Autodesk Fusion 360 part; units mm, degrees
note: some values were not read from the file. Chosen so that the rebuilt part matches the saved one: which face or edge a step refers to. Set by a fixed rule: which sketch regions a step uses.
(part 7 of 7)
  spline S202 degree 3 poles (37.6254, -69.5482) (37.6638, -69.7473) (37.7012, -69.9549) (37.7371, -70.1712) knots 0 0 0 0 1 1 1 1
  spline S203 degree 3 poles (37.7371, -70.1712) (37.8704, -70.972) (37.9841, -71.8901) (38.0568, -72.9254) knots 0 0 0 0 1 1 1 1
  arc A203 (36.6287, -73.6531) -> (38.0568, -72.9254) centre (0, 0) ccw
  spline S204 degree 3 poles (36.6287, -73.6531) (35.8338, -72.9858) (35.1579, -72.3541) (34.5883, -71.7756) knots 0 0 0 0 1 1 1 1
  spline S205 degree 3 poles (34.5883, -71.7756) (34.4345, -71.6193) (34.2885, -71.4671) (34.15, -71.319) knots 0 0 0 0 1 1 1 1
  arc A204 (34.15, -71.319) -> (33.6869, -71.2307) centre (33.8579, -71.5923) ccw
  arc A205 (32.2864, -71.8764) -> (33.6869, -71.2307) centre (0, 0) ccw
  arc A206 (32.2864, -71.8764) -> (32.0528, -72.2858) centre (32.4503, -72.2413) ccw
  spline S206 degree 3 poles (32.0528, -72.2858) (32.0754, -72.4873) (32.0964, -72.6972) (32.1152, -72.9157) knots 0 0 0 0 1 1 1 1
  spline S207 degree 3 poles (32.1152, -72.9157) (32.1852, -73.7245) (32.2266, -74.6487) (32.2178, -75.6865) knots 0 0 0 0 1 1 1 1
  arc A207 (30.737, -76.2999) -> (32.2178, -75.6865) centre (0, 0) ccw
  spline S208 degree 3 poles (30.737, -76.2999) (29.997, -75.5723) (29.3727, -74.8895) (28.8503, -74.2681) knots 0 0 0 0 1 1 1 1
  spline S209 degree 3 poles (28.8503, -74.2681) (28.7092, -74.1003) (28.5755, -73.937) (28.4491, -73.7785) knots 0 0 0 0 1 1 1 1
  arc A208 (28.4491, -73.7785) -> (27.9944, -73.6542) centre (28.1365, -74.0281) ccw
  arc A209 (26.5475, -74.188) -> (27.9944, -73.6542) centre (0, 0) ccw
  arc A210 (26.5475, -74.188) -> (26.2825, -74.5778) centre (26.6822, -74.5646) ccw
  spline S210 degree 3 poles (26.2825, -74.5778) (26.2892, -74.7805) (26.2937, -74.9914) (26.2953, -75.2107) knots 0 0 0 0 1 1 1 1
  spline S211 degree 3 poles (26.2953, -75.2107) (26.3016, -76.0225) (26.2704, -76.9471) (26.1802, -77.981) knots 0 0 0 0 1 1 1 1
  arc A211 (24.6558, -78.4763) -> (26.1802, -77.981) centre (0, 0) ccw
  spline S212 degree 3 poles (24.6558, -78.4763) (23.9752, -77.6928) (23.4064, -76.9632) (22.9343, -76.3027) knots 0 0 0 0 1 1 1 1
  spline S213 degree 3 poles (22.9343, -76.3027) (22.8068, -76.1243) (22.6864, -75.9511) (22.5728, -75.7832) knots 0 0 0 0 1 1 1 1
  arc A212 (22.5728, -75.7832) -> (22.1292, -75.6235) centre (22.2416, -76.0074) ccw
  arc A213 (20.6449, -76.0422) -> (22.1292, -75.6235) centre (0, 0) ccw
  arc A214 (20.6449, -76.0422) -> (20.3501, -76.41) centre (20.7497, -76.4282) ccw
  spline S214 degree 3 poles (20.3501, -76.41) (20.341, -76.6126) (20.3288, -76.8232) (20.3133, -77.0419) knots 0 0 0 0 1 1 1 1
  spline S215 degree 3 poles (20.3133, -77.0419) (20.2559, -77.8517) (20.1522, -78.771) (19.9812, -79.7947) knots 0 0 0 0 1 1 1 1
  arc A215 (18.4227, -80.1689) -> (19.9812, -79.7947) centre (0, 0) ccw
  spline S216 degree 3 poles (18.4227, -80.1689) (17.8055, -79.3344) (17.2958, -78.5624) (16.877, -77.8669) knots 0 0 0 0 1 1 1 1
  spline S217 degree 3 poles (16.877, -77.8669) (16.7639, -77.6791) (16.6574, -77.4969) (16.5573, -77.3206) knots 0 0 0 0 1 1 1 1
  arc A216 (16.5573, -77.3206) -> (16.1277, -77.1267) centre (16.2095, -77.5182) ccw
  arc A217 (14.6151, -77.4275) -> (16.1277, -77.1267) centre (0, 0) ccw
  arc A218 (14.6151, -77.4275) -> (14.2923, -77.7712) centre (14.6893, -77.8206) ccw
  spline S218 degree 3 poles (14.2923, -77.7712) (14.2673, -77.9723) (14.2387, -78.1814) (14.2061, -78.3982) knots 0 0 0 0 1 1 1 1
  spline S219 degree 3 poles (14.2061, -78.3982) (14.0853, -79.201) (13.9098, -80.1093) (13.659, -81.1164) knots 0 0 0 0 1 1 1 1
  arc A219 (12.0759, -81.3672) -> (13.659, -81.1164) centre (0, 0) ccw
  spline S220 degree 3 poles (12.0759, -81.3672) (11.5261, -80.4868) (11.0785, -79.6772) (10.7156, -78.951) knots 0 0 0 0 1 1 1 1
  spline S221 degree 3 poles (10.7156, -78.951) (10.6176, -78.7549) (10.5258, -78.5649) (10.4398, -78.3813) knots 0 0 0 0 1 1 1 1
  arc A220 (10.4398, -78.3813) -> (10.0267, -78.1543) centre (10.0776, -78.551) ccw
  arc A221 (8.4951, -78.3355) -> (10.0267, -78.1543) centre (0, 0) ccw
  arc A222 (8.4951, -78.3355) -> (8.1464, -78.6528) centre (8.5383, -78.7332) ccw
  spline S222 degree 3 poles (8.1464, -78.6528) (8.1057, -78.8514) (8.0608, -79.0575) (8.0112, -79.2711) knots 0 0 0 0 1 1 1 1
  spline S223 degree 3 poles (8.0112, -79.2711) (7.8278, -80.0619) (7.5816, -80.9537) (7.2526, -81.938) knots 0 0 0 0 1 1 1 1
  arc A223 (5.6547, -82.0638) -> (7.2526, -81.938) centre (0, 0) ccw
  spline S224 degree 3 poles (5.6547, -82.0638) (5.1757, -81.1431) (4.793, -80.3008) (4.4881, -79.5484) knots 0 0 0 0 1 1 1 1
  spline S225 degree 3 poles (4.4881, -79.5484) (4.4058, -79.3452) (4.3292, -79.1486) (4.2579, -78.9588) knots 0 0 0 0 1 1 1 1
  arc A224 (4.2579, -78.9588) -> (3.8638, -78.7) centre (3.8835, -79.0995) ccw
  arc A225 (2.3228, -78.7606) -> (3.8638, -78.7) centre (0, 0) ccw
  arc A226 (2.3228, -78.7606) -> (1.9503, -79.0495) centre (2.3346, -79.1604) ccw
  spline S226 degree 3 poles (1.9503, -79.0495) (1.8941, -79.2443) (1.8331, -79.4462) (1.767, -79.6553) knots 0 0 0 0 1 1 1 1
  spline S227 degree 3 poles (1.767, -79.6553) (1.5221, -80.4293) (1.2067, -81.299) (0.8014, -82.2545) knots 0 0 0 0 1 1 1 1
  arc A227 (-0.8014, -82.2545) -> (0.8014, -82.2545) centre (0, 0) ccw
  spline S228 degree 3 poles (-0.8014, -82.2545) (-1.2067, -81.299) (-1.5221, -80.4293) (-1.767, -79.6553) knots 0 0 0 0 1 1 1 1
  spline S229 degree 3 poles (-1.767, -79.6553) (-1.8331, -79.4462) (-1.8941, -79.2443) (-1.9503, -79.0495) knots 0 0 0 0 1 1 1 1
  arc A228 (-1.9503, -79.0495) -> (-2.3228, -78.7606) centre (-2.3346, -79.1604) ccw
  arc A229 (-3.8638, -78.7) -> (-2.3228, -78.7606) centre (0, 0) ccw
  arc A230 (-3.8638, -78.7) -> (-4.2579, -78.9588) centre (-3.8835, -79.0995) ccw
  spline S230 degree 3 poles (-4.2579, -78.9588) (-4.3292, -79.1486) (-4.4058, -79.3452) (-4.4881, -79.5484) knots 0 0 0 0 1 1 1 1
  spline S231 degree 3 poles (-4.4881, -79.5484) (-4.793, -80.3008) (-5.1757, -81.1431) (-5.6547, -82.0638) knots 0 0 0 0 1 1 1 1
  arc A231 (-7.2526, -81.938) -> (-5.6547, -82.0638) centre (0, 0) ccw
  spline S232 degree 3 poles (-7.2526, -81.938) (-7.5816, -80.9537) (-7.8278, -80.0619) (-8.0112, -79.2711) knots 0 0 0 0 1 1 1 1
  spline S233 degree 3 poles (-8.0112, -79.2711) (-8.0608, -79.0575) (-8.1057, -78.8514) (-8.1464, -78.6528) knots 0 0 0 0 1 1 1 1
  arc A232 (-8.1464, -78.6528) -> (-8.4951, -78.3355) centre (-8.5383, -78.7332) ccw
  arc A233 (-10.0267, -78.1543) -> (-8.4951, -78.3355) centre (0, 0) ccw
  arc A234 (-10.0267, -78.1543) -> (-10.4398, -78.3813) centre (-10.0776, -78.551) ccw
  spline S234 degree 3 poles (-10.4398, -78.3813) (-10.5258, -78.5649) (-10.6176, -78.7549) (-10.7156, -78.951) knots 0 0 0 0 1 1 1 1
  spline S235 degree 3 poles (-10.7156, -78.951) (-11.0785, -79.6772) (-11.5261, -80.4868) (-12.0759, -81.3672) knots 0 0 0 0 1 1 1 1
  arc A235 (-13.659, -81.1164) -> (-12.0759, -81.3672) centre (0, 0) ccw
  spline S236 degree 3 poles (-13.659, -81.1164) (-13.9098, -80.1093) (-14.0853, -79.201) (-14.2061, -78.3982) knots 0 0 0 0 1 1 1 1
  spline S237 degree 3 poles (-14.2061, -78.3982) (-14.2387, -78.1814) (-14.2673, -77.9723) (-14.2923, -77.7712) knots 0 0 0 0 1 1 1 1
  arc A236 (-14.2923, -77.7712) -> (-14.6151, -77.4275) centre (-14.6893, -77.8206) ccw
  arc A237 (-16.1277, -77.1267) -> (-14.6151, -77.4275) centre (0, 0) ccw
  arc A238 (-16.1277, -77.1267) -> (-16.5573, -77.3206) centre (-16.2095, -77.5182) ccw
  spline S238 degree 3 poles (-16.5573, -77.3206) (-16.6574, -77.4969) (-16.7639, -77.6791) (-16.877, -77.8669) knots 0 0 0 0 1 1 1 1
  spline S239 degree 3 poles (-16.877, -77.8669) (-17.2958, -78.5624) (-17.8055, -79.3344) (-18.4227, -80.1689) knots 0 0 0 0 1 1 1 1
  arc A239 (-19.9812, -79.7947) -> (-18.4227, -80.1689) centre (0, 0) ccw
  spline S240 degree 3 poles (-19.9812, -79.7947) (-20.1522, -78.771) (-20.2559, -77.8517) (-20.3133, -77.0419) knots 0 0 0 0 1 1 1 1
  spline S241 degree 3 poles (-20.3133, -77.0419) (-20.3288, -76.8232) (-20.341, -76.6126) (-20.3501, -76.41) knots 0 0 0 0 1 1 1 1
  arc A240 (-20.3501, -76.41) -> (-20.6449, -76.0422) centre (-20.7497, -76.4282) ccw
  arc A241 (-22.1292, -75.6235) -> (-20.6449, -76.0422) centre (0, 0) ccw
  arc A242 (-22.1292, -75.6235) -> (-22.5728, -75.7832) centre (-22.2416, -76.0074) ccw
  spline S242 degree 3 poles (-22.5728, -75.7832) (-22.6864, -75.9511) (-22.8068, -76.1243) (-22.9343, -76.3027) knots 0 0 0 0 1 1 1 1
  spline S243 degree 3 poles (-22.9343, -76.3027) (-23.4064, -76.9632) (-23.9752, -77.6928) (-24.6558, -78.4763) knots 0 0 0 0 1 1 1 1
  arc A243 (-26.1802, -77.981) -> (-24.6558, -78.4763) centre (0, 0) ccw
  spline S244 degree 3 poles (-26.1802, -77.981) (-26.2704, -76.9471) (-26.3016, -76.0225) (-26.2953, -75.2107) knots 0 0 0 0 1 1 1 1
  spline S245 degree 3 poles (-26.2953, -75.2107) (-26.2937, -74.9914) (-26.2892, -74.7805) (-26.2825, -74.5778) knots 0 0 0 0 1 1 1 1
  arc A244 (-26.2825, -74.5778) -> (-26.5475, -74.188) centre (-26.6822, -74.5646) ccw
  arc A245 (-27.9944, -73.6542) -> (-26.5475, -74.188) centre (0, 0) ccw
  arc A246 (-27.9944, -73.6542) -> (-28.4491, -73.7785) centre (-28.1365, -74.0281) ccw
  spline S246 degree 3 poles (-28.4491, -73.7785) (-28.5755, -73.937) (-28.7092, -74.1003) (-28.8503, -74.2681) knots 0 0 0 0 1 1 1 1
  spline S247 degree 3 poles (-28.8503, -74.2681) (-29.3727, -74.8895) (-29.997, -75.5723) (-30.737, -76.2999) knots 0 0 0 0 1 1 1 1
  arc A247 (-32.2178, -75.6865) -> (-30.737, -76.2999) centre (0, 0) ccw
  spline S248 degree 3 poles (-32.2178, -75.6865) (-32.2266, -74.6487) (-32.1852, -73.7245) (-32.1152, -72.9157) knots 0 0 0 0 1 1 1 1
  spline S249 degree 3 poles (-32.1152, -72.9157) (-32.0964, -72.6972) (-32.0754, -72.4873) (-32.0528, -72.2858) knots 0 0 0 0 1 1 1 1
  arc A248 (-32.0528, -72.2858) -> (-32.2864, -71.8764) centre (-32.4503, -72.2413) ccw
  arc A249 (-33.6869, -71.2307) -> (-32.2864, -71.8764) centre (0, 0) ccw
  arc A250 (-33.6869, -71.2307) -> (-34.15, -71.319) centre (-33.8579, -71.5923) ccw
  spline S250 degree 3 poles (-34.15, -71.319) (-34.2885, -71.4671) (-34.4345, -71.6193) (-34.5883, -71.7756) knots 0 0 0 0 1 1 1 1
  spline S251 degree 3 poles (-34.5883, -71.7756) (-35.1579, -72.3541) (-35.8338, -72.9858) (-36.6287, -73.6531) knots 0 0 0 0 1 1 1 1
  arc A251 (-38.0568, -72.9254) -> (-36.6287, -73.6531) centre (0, 0) ccw
  spline S252 degree 3 poles (-38.0568, -72.9254) (-37.9841, -71.8901) (-37.8704, -70.972) (-37.7371, -70.1712) knots 0 0 0 0 1 1 1 1
  spline S253 degree 3 poles (-37.7371, -70.1712) (-37.7012, -69.9549) (-37.6638, -69.7473) (-37.6254, -69.5482) knots 0 0 0 0 1 1 1 1
  arc A252 (-37.6254, -69.5482) -> (-37.8262, -69.1217) centre (-38.0182, -69.4726) ccw
  arc A253 (-39.1718, -68.3681) -> (-37.8262, -69.1217) centre (0, 0) ccw
  arc A254 (-39.1718, -68.3681) -> (-39.6403, -68.4198) centre (-39.3706, -68.7152) ccw
  spline S254 degree 3 poles (-39.6403, -68.4198) (-39.79, -68.5565) (-39.9475, -68.6969) (-40.1132, -68.8406) knots 0 0 0 0 1 1 1 1
  spline S255 degree 3 poles (-40.1132, -68.8406) (-40.7264, -69.3726) (-41.4498, -69.9493) (-42.2945, -70.5522) knots 0 0 0 0 1 1 1 1
  arc A255 (-43.6612, -69.7147) -> (-42.2945, -70.5522) centre (0, 0) ccw
  spline S256 degree 3 poles (-43.6612, -69.7147) (-43.5075, -68.6883) (-43.322, -67.7819) (-43.1264, -66.9941) knots 0 0 0 0 1 1 1 1
  spline S257 degree 3 poles (-43.1264, -66.9941) (-43.0736, -66.7812) (-43.02, -66.5772) (-42.9661, -66.3817) knots 0 0 0 0 1 1 1 1
  arc A256 (-42.9661, -66.3817) -> (-43.1328, -65.9408) centre (-43.3518, -66.2755) ccw
  arc A257 (-44.4151, -65.084) -> (-43.1328, -65.9408) centre (0, 0) ccw
  arc A258 (-44.4151, -65.084) -> (-44.8863, -65.0987) centre (-44.6406, -65.4144) ccw
  spline S258 degree 3 poles (-44.8863, -65.0987) (-45.0463, -65.2233) (-45.2143, -65.3508) (-45.3907, -65.4811) knots 0 0 0 0 1 1 1 1
  spline S259 degree 3 poles (-45.3907, -65.4811) (-46.0437, -65.9633) (-46.8101, -66.4815) (-47.6996, -67.0163) knots 0 0 0 0 1 1 1 1
  arc A259 (-48.9963, -66.0742) -> (-47.6996, -67.0163) centre (0, 0) ccw
  spline S260 degree 3 poles (-48.9963, -66.0742) (-48.7626, -65.063) (-48.5066, -64.174) (-48.2497, -63.4039) knots 0 0 0 0 1 1 1 1
  spline S261 degree 3 poles (-48.2497, -63.4039) (-48.1804, -63.1959) (-48.111, -62.9966) (-48.0419, -62.806) knots 0 0 0 0 1 1 1 1
  arc A260 (-48.0419, -62.806) -> (-48.1735, -62.3533) centre (-48.418, -62.6699) ccw
  arc A261 (-49.3846, -61.3986) -> (-48.1735, -62.3533) centre (0, 0) ccw
  arc A262 (-49.3846, -61.3986) -> (-49.8555, -61.3763) centre (-49.6353, -61.7102) ccw
  spline S262 degree 3 poles (-49.8555, -61.3763) (-50.0247, -61.4879) (-50.2023, -61.6019) (-50.3883, -61.7179) knots 0 0 0 0 1 1 1 1
  spline S263 degree 3 poles (-50.3883, -61.7179) (-51.0772, -62.1475) (-51.8819, -62.6039) (-52.8106, -63.0673) knots 0 0 0 0 1 1 1 1
  arc A263 (-54.0294, -62.0263) -> (-52.8106, -63.0673) centre (0, 0) ccw
  spline S264 degree 3 poles (-54.0294, -62.0263) (-53.717, -61.0366) (-53.3921, -60.1704) (-53.0756, -59.4228) knots 0 0 0 0 1 1 1 1
  spline S265 degree 3 poles (-53.0756, -59.4228) (-52.9901, -59.2209) (-52.9053, -59.0277) (-52.8215, -58.8431) knots 0 0 0 0 1 1 1 1
  arc A264 (-52.8215, -58.8431) -> (-52.9172, -58.3815) centre (-53.1858, -58.6778) ccw
  arc A265 (-54.0497, -57.3346) -> (-52.9172, -58.3815) centre (0, 0) ccw
  arc A266 (-54.0497, -57.3346) -> (-54.5174, -57.2755) centre (-54.324, -57.6257) ccw
  spline S266 degree 3 poles (-54.5174, -57.2755) (-54.6948, -57.3735) (-54.8807, -57.4732) (-55.0753, -57.5742) knots 0 0 0 0 1 1 1 1
  spline S267 degree 3 poles (-55.0753, -57.5742) (-55.7958, -57.9484) (-56.6338, -58.3403) (-57.596, -58.7294) knots 0 0 0 0 1 1 1 1
  arc A267 (-58.7294, -57.596) -> (-57.596, -58.7294) centre (0, 0) ccw
  spline S268 degree 3 poles (-58.7294, -57.596) (-58.3403, -56.6338) (-57.9484, -55.7958) (-57.5742, -55.0753) knots 0 0 0 0 1 1 1 1
  spline S269 degree 3 poles (-57.5742, -55.0753) (-57.4732, -54.8807) (-57.3735, -54.6948) (-57.2755, -54.5174) knots 0 0 0 0 1 1 1 1
  arc A268 (-57.2755, -54.5174) -> (-57.3346, -54.0497) centre (-57.6257, -54.324) ccw
  arc A269 (-58.3815, -52.9172) -> (-57.3346, -54.0497) centre (0, 0) ccw
  arc A270 (-58.3815, -52.9172) -> (-58.8431, -52.8215) centre (-58.6778, -53.1858) ccw
  spline S270 degree 3 poles (-58.8431, -52.8215) (-59.0277, -52.9053) (-59.2209, -52.9901) (-59.4228, -53.0756) knots 0 0 0 0 1 1 1 1
  spline S271 degree 3 poles (-59.4228, -53.0756) (-60.1704, -53.3921) (-61.0366, -53.717) (-62.0263, -54.0294) knots 0 0 0 0 1 1 1 1
  arc A271 (-63.0673, -52.8106) -> (-62.0263, -54.0294) centre (0, 0) ccw
  spline S272 degree 3 poles (-63.0673, -52.8106) (-62.6039, -51.8819) (-62.1475, -51.0772) (-61.7179, -50.3883) knots 0 0 0 0 1 1 1 1
  spline S273 degree 3 poles (-61.7179, -50.3883) (-61.6019, -50.2023) (-61.4879, -50.0247) (-61.3763, -49.8555) knots 0 0 0 0 1 1 1 1
  arc A272 (-61.3763, -49.8555) -> (-61.3986, -49.3846) centre (-61.7102, -49.6353) ccw
  arc A273 (-62.3533, -48.1735) -> (-61.3986, -49.3846) centre (0, 0) ccw
  arc A274 (-62.3533, -48.1735) -> (-62.806, -48.0419) centre (-62.6699, -48.418) ccw
  spline S274 degree 3 poles (-62.806, -48.0419) (-62.9966, -48.111) (-63.1959, -48.1804) (-63.4039, -48.2497) knots 0 0 0 0 1 1 1 1
  spline S275 degree 3 poles (-63.4039, -48.2497) (-64.174, -48.5066) (-65.063, -48.7626) (-66.0742, -48.9963) knots 0 0 0 0 1 1 1 1
  arc A275 (-67.0163, -47.6996) -> (-66.0742, -48.9963) centre (0, 0) ccw
  spline S276 degree 3 poles (-67.0163, -47.6996) (-66.4815, -46.8101) (-65.9633, -46.0437) (-65.4811, -45.3907) knots 0 0 0 0 1 1 1 1
  spline S277 degree 3 poles (-65.4811, -45.3907) (-65.3508, -45.2143) (-65.2233, -45.0463) (-65.0987, -44.8863) knots 0 0 0 0 1 1 1 1
  arc A276 (-65.0987, -44.8863) -> (-65.084, -44.4151) centre (-65.4144, -44.6406) ccw
  arc A277 (-65.9408, -43.1328) -> (-65.084, -44.4151) centre (0, 0) ccw
  arc A278 (-65.9408, -43.1328) -> (-66.3817, -42.9661) centre (-66.2755, -43.3518) ccw
  spline S278 degree 3 poles (-66.3817, -42.9661) (-66.5772, -43.02) (-66.7812, -43.0736) (-66.9941, -43.1264) knots 0 0 0 0 1 1 1 1
  spline S279 degree 3 poles (-66.9941, -43.1264) (-67.7819, -43.322) (-68.6883, -43.5075) (-69.7147, -43.6612) knots 0 0 0 0 1 1 1 1
  arc A279 (-70.5522, -42.2945) -> (-69.7147, -43.6612) centre (0, 0) ccw
  spline S280 degree 3 poles (-70.5522, -42.2945) (-69.9493, -41.4498) (-69.3726, -40.7264) (-68.8406, -40.1132) knots 0 0 0 0 1 1 1 1
  spline S281 degree 3 poles (-68.8406, -40.1132) (-68.6969, -39.9475) (-68.5565, -39.79) (-68.4198, -39.6403) knots 0 0 0 0 1 1 1 1
  arc A280 (-68.4198, -39.6403) -> (-68.3681, -39.1718) centre (-68.7152, -39.3706) ccw
  arc A281 (-69.1217, -37.8262) -> (-68.3681, -39.1718) centre (0, 0) ccw
  arc A282 (-69.1217, -37.8262) -> (-69.5482, -37.6254) centre (-69.4726, -38.0182) ccw
  spline S282 degree 3 poles (-69.5482, -37.6254) (-69.7473, -37.6638) (-69.9549, -37.7012) (-70.1712, -37.7371) knots 0 0 0 0 1 1 1 1
  spline S283 degree 3 poles (-70.1712, -37.7371) (-70.972, -37.8704) (-71.8901, -37.9841) (-72.9254, -38.0568) knots 0 0 0 0 1 1 1 1
  arc A283 (-73.6531, -36.6287) -> (-72.9254, -38.0568) centre (0, 0) ccw
  spline S284 degree 3 poles (-73.6531, -36.6287) (-72.9858, -35.8338) (-72.3541, -35.1579) (-71.7756, -34.5883) knots 0 0 0 0 1 1 1 1
  spline S285 degree 3 poles (-71.7756, -34.5883) (-71.6193, -34.4345) (-71.4671, -34.2885) (-71.319, -34.15) knots 0 0 0 0 1 1 1 1
  arc A284 (-71.319, -34.15) -> (-71.2307, -33.6869) centre (-71.5923, -33.8579) ccw
  arc A285 (-71.8764, -32.2864) -> (-71.2307, -33.6869) centre (0, 0) ccw
  arc A286 (-71.8764, -32.2864) -> (-72.2858, -32.0528) centre (-72.2413, -32.4503) ccw
  spline S286 degree 3 poles (-72.2858, -32.0528) (-72.4873, -32.0754) (-72.6972, -32.0964) (-72.9157, -32.1152) knots 0 0 0 0 1 1 1 1
  spline S287 degree 3 poles (-72.9157, -32.1152) (-73.7245, -32.1852) (-74.6487, -32.2266) (-75.6865, -32.2178) knots 0 0 0 0 1 1 1 1
  arc A287 (-76.2999, -30.737) -> (-75.6865, -32.2178) centre (0, 0) ccw
  spline S288 degree 3 poles (-76.2999, -30.737) (-75.5723, -29.997) (-74.8895, -29.3727) (-74.2681, -28.8503) knots 0 0 0 0 1 1 1 1
  spline S289 degree 3 poles (-74.2681, -28.8503) (-74.1003, -28.7092) (-73.937, -28.5755) (-73.7785, -28.4491) knots 0 0 0 0 1 1 1 1
  arc A288 (-73.7785, -28.4491) -> (-73.6542, -27.9944) centre (-74.0281, -28.1365) ccw
  arc A289 (-74.188, -26.5475) -> (-73.6542, -27.9944) centre (0, 0) ccw
  arc A290 (-74.188, -26.5475) -> (-74.5778, -26.2825) centre (-74.5646, -26.6822) ccw
  spline S290 degree 3 poles (-74.5778, -26.2825) (-74.7805, -26.2892) (-74.9914, -26.2937) (-75.2107, -26.2953) knots 0 0 0 0 1 1 1 1
  spline S291 degree 3 poles (-75.2107, -26.2953) (-76.0225, -26.3016) (-76.9471, -26.2704) (-77.981, -26.1802) knots 0 0 0 0 1 1 1 1
  arc A291 (-78.4763, -24.6558) -> (-77.981, -26.1802) centre (0, 0) ccw
  spline S292 degree 3 poles (-78.4763, -24.6558) (-77.6928, -23.9752) (-76.9632, -23.4064) (-76.3027, -22.9343) knots 0 0 0 0 1 1 1 1
  spline S293 degree 3 poles (-76.3027, -22.9343) (-76.1243, -22.8068) (-75.9511, -22.6864) (-75.7832, -22.5728) knots 0 0 0 0 1 1 1 1
  arc A292 (-75.7832, -22.5728) -> (-75.6235, -22.1292) centre (-76.0074, -22.2416) ccw
  arc A293 (-76.0422, -20.6449) -> (-75.6235, -22.1292) centre (0, 0) ccw
  arc A294 (-76.0422, -20.6449) -> (-76.41, -20.3501) centre (-76.4282, -20.7497) ccw
  spline S294 degree 3 poles (-76.41, -20.3501) (-76.6126, -20.341) (-76.8232, -20.3288) (-77.0419, -20.3133) knots 0 0 0 0 1 1 1 1
  spline S295 degree 3 poles (-77.0419, -20.3133) (-77.8517, -20.2559) (-78.771, -20.1522) (-79.7947, -19.9812) knots 0 0 0 0 1 1 1 1
  arc A295 (-80.1689, -18.4227) -> (-79.7947, -19.9812) centre (0, 0) ccw
  spline S296 degree 3 poles (-80.1689, -18.4227) (-79.3344, -17.8055) (-78.5624, -17.2958) (-77.8669, -16.877) knots 0 0 0 0 1 1 1 1
  spline S297 degree 3 poles (-77.8669, -16.877) (-77.6791, -16.7639) (-77.4969, -16.6574) (-77.3206, -16.5573) knots 0 0 0 0 1 1 1 1
  arc A296 (-77.3206, -16.5573) -> (-77.1267, -16.1277) centre (-77.5182, -16.2095) ccw
  arc A297 (-77.4275, -14.6151) -> (-77.1267, -16.1277) centre (0, 0) ccw
  arc A298 (-77.4275, -14.6151) -> (-77.7712, -14.2923) centre (-77.8206, -14.6893) ccw
  spline S298 degree 3 poles (-77.7712, -14.2923) (-77.9723, -14.2673) (-78.1814, -14.2387) (-78.3982, -14.2061) knots 0 0 0 0 1 1 1 1
  spline S299 degree 3 poles (-78.3982, -14.2061) (-79.201, -14.0853) (-80.1093, -13.9098) (-81.1164, -13.659) knots 0 0 0 0 1 1 1 1
  arc A299 (-81.3672, -12.0759) -> (-81.1164, -13.659) centre (0, 0) ccw
  spline S300 degree 3 poles (-81.3672, -12.0759) (-80.4868, -11.5261) (-79.6772, -11.0785) (-78.951, -10.7156) knots 0 0 0 0 1 1 1 1
  spline S301 degree 3 poles (-78.951, -10.7156) (-78.7549, -10.6176) (-78.5649, -10.5258) (-78.3813, -10.4398) knots 0 0 0 0 1 1 1 1
  arc A300 (-78.3813, -10.4398) -> (-78.1543, -10.0267) centre (-78.551, -10.0776) ccw
  arc A301 (-78.3355, -8.4951) -> (-78.1543, -10.0267) centre (0, 0) ccw
  arc A302 (-78.3355, -8.4951) -> (-78.6528, -8.1464) centre (-78.7332, -8.5383) ccw
  spline S302 degree 3 poles (-78.6528, -8.1464) (-78.8514, -8.1057) (-79.0575, -8.0608) (-79.2711, -8.0112) knots 0 0 0 0 1 1 1 1
  spline S303 degree 3 poles (-79.2711, -8.0112) (-80.0619, -7.8278) (-80.9537, -7.5816) (-81.938, -7.2526) knots 0 0 0 0 1 1 1 1
  arc A303 (-82.0638, -5.6547) -> (-81.938, -7.2526) centre (0, 0) ccw
  spline S304 degree 3 poles (-82.0638, -5.6547) (-81.1431, -5.1757) (-80.3008, -4.793) (-79.5484, -4.4881) knots 0 0 0 0 1 1 1 1
  spline S305 degree 3 poles (-79.5484, -4.4881) (-79.3452, -4.4058) (-79.1486, -4.3292) (-78.9588, -4.2579) knots 0 0 0 0 1 1 1 1
  arc A304 (-78.9588, -4.2579) -> (-78.7, -3.8638) centre (-79.0995, -3.8835) ccw
  arc A305 (-78.7606, -2.3228) -> (-78.7, -3.8638) centre (0, 0) ccw
  arc A306 (-78.7606, -2.3228) -> (-79.0495, -1.9503) centre (-79.1604, -2.3346) ccw
  spline S306 degree 3 poles (-79.0495, -1.9503) (-79.2443, -1.8941) (-79.4462, -1.8331) (-79.6553, -1.767) knots 0 0 0 0 1 1 1 1
  spline S307 degree 3 poles (-79.6553, -1.767) (-80.4293, -1.5221) (-81.299, -1.2067) (-82.2545, -0.8014) knots 0 0 0 0 1 1 1 1
  arc A307 (-82.2545, 0.8014) -> (-82.2545, -0.8014) centre (0, 0) ccw
  spline S308 degree 3 poles (-82.2545, 0.8014) (-81.299, 1.2067) (-80.4293, 1.5221) (-79.6553, 1.767) knots 0 0 0 0 1 1 1 1
  spline S309 degree 3 poles (-79.6553, 1.767) (-79.4462, 1.8331) (-79.2443, 1.8941) (-79.0495, 1.9503) knots 0 0 0 0 1 1 1 1
  arc A308 (-79.0495, 1.9503) -> (-78.7606, 2.3228) centre (-79.1604, 2.3346) ccw
  arc A309 (-78.7, 3.8638) -> (-78.7606, 2.3228) centre (0, 0) ccw
  arc A310 (-78.7, 3.8638) -> (-78.9588, 4.2579) centre (-79.0995, 3.8835) ccw
  spline S310 degree 3 poles (-78.9588, 4.2579) (-79.1486, 4.3292) (-79.3452, 4.4058) (-79.5484, 4.4881) knots 0 0 0 0 1 1 1 1
  spline S311 degree 3 poles (-79.5484, 4.4881) (-80.3008, 4.793) (-81.1431, 5.1757) (-82.0638, 5.6547) knots 0 0 0 0 1 1 1 1
  arc A311 (-81.938, 7.2526) -> (-82.0638, 5.6547) centre (0, 0) ccw
  spline S312 degree 3 poles (-81.938, 7.2526) (-80.9537, 7.5816) (-80.0619, 7.8278) (-79.2711, 8.0112) knots 0 0 0 0 1 1 1 1
  spline S313 degree 3 poles (-79.2711, 8.0112) (-79.0575, 8.0608) (-78.8514, 8.1057) (-78.6528, 8.1464) knots 0 0 0 0 1 1 1 1
  arc A312 (-78.6528, 8.1464) -> (-78.3355, 8.4951) centre (-78.7332, 8.5383) ccw
  arc A313 (-78.1543, 10.0267) -> (-78.3355, 8.4951) centre (0, 0) ccw
  arc A314 (-78.1543, 10.0267) -> (-78.3813, 10.4398) centre (-78.551, 10.0776) ccw
  spline S314 degree 3 poles (-78.3813, 10.4398) (-78.5649, 10.5258) (-78.7549, 10.6176) (-78.951, 10.7156) knots 0 0 0 0 1 1 1 1
  spline S315 degree 3 poles (-78.951, 10.7156) (-79.6772, 11.0785) (-80.4868, 11.5261) (-81.3672, 12.0759) knots 0 0 0 0 1 1 1 1
  arc A315 (-81.1164, 13.659) -> (-81.3672, 12.0759) centre (0, 0) ccw
  spline S316 degree 3 poles (-81.1164, 13.659) (-80.1093, 13.9098) (-79.201, 14.0853) (-78.3982, 14.2061) knots 0 0 0 0 1 1 1 1
  spline S317 degree 3 poles (-78.3982, 14.2061) (-78.1814, 14.2387) (-77.9723, 14.2673) (-77.7712, 14.2923) knots 0 0 0 0 1 1 1 1
  arc A316 (-77.7712, 14.2923) -> (-77.4275, 14.6151) centre (-77.8206, 14.6893) ccw
  arc A317 (-77.1267, 16.1277) -> (-77.4275, 14.6151) centre (0, 0) ccw
  arc A318 (-77.1267, 16.1277) -> (-77.3206, 16.5573) centre (-77.5182, 16.2095) ccw
  spline S318 degree 3 poles (-77.3206, 16.5573) (-77.4969, 16.6574) (-77.6791, 16.7639) (-77.8669, 16.877) knots 0 0 0 0 1 1 1 1
  spline S319 degree 3 poles (-77.8669, 16.877) (-78.5624, 17.2958) (-79.3344, 17.8055) (-80.1689, 18.4227) knots 0 0 0 0 1 1 1 1
  arc A319 (-79.7947, 19.9812) -> (-80.1689, 18.4227) centre (0, 0) ccw
  circle A320 centre (0, 0) radius 92.5
extrude "Extrude3''" add sketch "Sketch15" against normal blind 24 contours A320 A321 | A320 A323 | A320 A322 picked at (-0.0821, 85.8471) picked at (74.5605, -42.5553) picked at (-74.1888, -43.1909) bodies 3 in component "Internal Gear (80 teeth)"
mirror "MirrorComponent2" about plane through (0, 0, 0) normal (0, 0, 1) of bodies 7 makes body 9 in component "Component15(Mirror)"
sketch "Sketch24" plane through (0, 0, 0) normal (0, 1, 0) x (1, 0, 0)
  circle A0 centre (0, 0) radius 92.5
  circle A1 centre (0, 0) radius 92.5
  line L0 (-72.1204, 57.9215) -> (-72.1204, 110)
  line L1 (-72.1204, 110) -> (0, 110)
  line L2 (0, 110) -> (0, 100)
  line L3 (72.1204, 57.9215) -> (72.1204, 110)
  line L4 (72.1204, 110) -> (0, 110)
component "Spur Gear (20 teeth)" placed x (0.996195, 0, 0.087156) y (0, 1, 0) z (-0.087156, 0, 0.996195) at (41.6795, 0, 43.1604)
component "Spur Gear (40 teeth)" placed x (1, 0, 0) y (0, 1, 0) z (0, 0, 1) at (0, 0, 0)
component "Internal Gear (80 teeth)" placed x (1, 0, 0) y (0, 1, 0) z (0, 0, 1) at (0, 0, 0)
component "Component" placed x (1, 0, 0) y (0, 1, 0) z (0, 0, 1) at (0, 0, 0)
component "Component'" placed x (1, 0, 0) y (0, 1, 0) z (0, 0, 1) at (0, 0, 0)
component "Component''" placed x (1, 0, 0) y (0, 1, 0) z (0, 0, 1) at (0, 0, 0)
component "Component'''" placed x (1, 0, 0) y (0, 1, 0) z (0, 0, 1) at (0, 0, 0)
component "Component15(Mirror)" placed x (1, 0, 0) y (0, -1, 0) z (0, 0, -1) at (0, 12, 0)
hidden bodies 6
equation "d108 = -8 mm - 16 mm"
